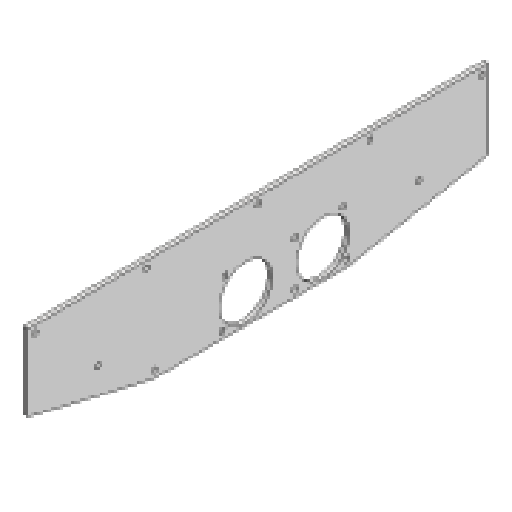
# Autodesk Inventor part: InsideChassiPlate3.0
Saved by Autodesk Inventor 2023 (Build 270158000, 158)
## iProperties
Created: 2022-09-18
Part Number: InsideChassiPlate3.0
Material: Generic
Document SubType Name: Modeling
Designer: deli
Density: 1 g/cm^3
Appearance: Default
Mass: 76.7316 g
Surface Area: 518.075 cm^2
Volume: 76.7316 cm^3
Author: deli
Autodesk Inventor part; units mm, degrees
ref_plane "YZ Plane" through (0, 0, 0) normal (1, 0, 0) x (0, 1, 0)
ref_plane "XZ Plane" through (0, 0, 0) normal (0, 1, 0) x (-1, 0, 0)
ref_plane "XY Plane" through (0, 0, 0) normal (0, 0, 1) x (1, 0, 0)
sketch "Sketch1" plane through (0, 0, 0) normal (1, 0, 0) x (0, 1, 0)
  line L0 (253.267, 23.7536) -> (253.267, 96.2747) projected
  line L1 (253.267, 96.2747) -> (174.6274, 96.2747) projected
  line L2 (174.6274, 96.2747) -> (153.402, 6.7905) projected
  arc A0 (153.402, 6.7905) -> (153.267, 5.6365) centre (158.267, 5.6365) ccw projected
  line L3 (153.267, 5.6365) -> (153.267, -132.1707) projected
  arc A1 (153.267, -132.1707) -> (153.3544, -133.1015) centre (158.267, -132.1707) ccw projected
  line L4 (153.3544, -133.1015) -> (172.4208, -233.7253) projected
  line L5 (172.4208, -233.7253) -> (251.0603, -233.7253) projected
  line L6 (251.0603, -233.7253) -> (579.954, -176.0645) projected
  arc A2 (579.954, -176.0645) -> (580.5697, -168.344) centre (579.2633, -172.1246) ccw projected
  line L7 (580.5697, -168.344) -> (526.3406, -149.6042) projected
  arc A3 (525.9265, -149.4053) -> (526.3406, -149.6042) centre (526.9939, -147.7139) ccw projected
  line L8 (525.9265, -149.4053) -> (254.1996, 22.0622) projected
  arc A4 (253.267, 23.7536) -> (254.1996, 22.0622) centre (255.267, 23.7536) ccw projected
  circle A5 centre (508.1, -149.9808) radius 1.5 projected
  circle A6 centre (393.9306, -77.9366) radius 1.5 projected
  circle A7 centre (279.7613, -5.8925) radius 1.5 projected
  circle A8 centre (579.2633, -172.1246) radius 1.6 projected
  circle A9 centre (224.267, -228.7253) radius 2 projected
  circle A10 centre (224.267, 11.2747) radius 2 projected
  circle A11 centre (191.6977, -44.8173) radius 2 projected
  circle A12 centre (192.186, -129.5748) radius 2 projected
  circle A13 centre (181.267, 46.2747) radius 2 projected
  circle A14 centre (181.267, -183.7253) radius 2 projected
  circle A15 centre (174.017, -59.9155) radius 7 projected
  circle A16 centre (174.017, -115.0681) radius 7 projected
  circle A17 centre (190.1509, -94.9992) radius 2 projected
  circle A18 centre (157.883, -94.9992) radius 2 projected
  circle A19 centre (158.267, -42.8128) radius 2 projected
  circle A20 centre (224.267, 91.2747) radius 2 projected
  circle A21 centre (224.267, -148.7253) radius 2 projected
  circle A22 centre (224.267, -68.7253) radius 2 projected
  circle A23 centre (158.267, 5.6365) radius 2 projected
  circle A24 centre (158.267, -132.1707) radius 2 projected
  line L9 (229.267, 96.2747) -> (229.267, -233.7253)
  circle A25 centre (174.017, -59.9155) radius 19
  circle A26 centre (174.017, -115.0681) radius 19
  dimension "d14" = 5
  dimension "d15" = 38
  constraints: 2 centre point, 2 coincident, 2 end point, 2 point on line, 1 equal radius, 1 vertical
  measures "d14" distance from line of A10.centre L9
  measures "d15" diameter of A25
extrude "Extrusion1" add sketch "Sketch1" along normal blind 3.175 contours L9 L5 L4 A1 L3 A0 L2 L1
body "Solid1"
